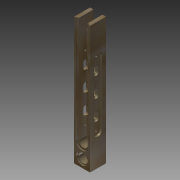
# Autodesk Inventor part: 13_1087_009
Saved by Autodesk Inventor 2014 (Build 180170000, 170)
## iProperties
Created: 2013-08-07
Part Number: 13_1087_009
Material: PVC, hart
Document SubType Name: Modeling
Designer: vogel
Density: 1.4 g/cm^3
Appearance: Sperrholz - verwittert
Author: vogel
Autodesk Inventor part; units mm, degrees
ref_plane "YZ Plane" through (0, 0, 0) normal (1, 0, 0) x (0, 1, 0)
ref_plane "XZ Plane" through (0, 0, 0) normal (0, 1, 0) x (-1, 0, 0)
sketch "Skizze1" plane through (0, 0, 0) normal (0, 0, 1) x (1, 0, 0)
  line L0 (-9.8, 0) -> (9.8, 0) projected
  line L1 (0, -9.8) -> (0, 9.8) projected
  line L2 (-7, 7) -> (7, 7)
  line L3 (7, 7) -> (7, -7)
  line L4 (7, -7) -> (-7, -7)
  line L5 (-7, -7) -> (-7, 7)
  point P0 (0, 0)
  dimension "d0" = 14
  dimension "d1" = 14
  constraints: 8 end point, 2 parallel, 1 horizontal, 1 perpendicular, 2 other
  measures "d0" distance of L2.start L2.end
  measures "d1" distance of L4.end L2.start
extrude "Extrusion1" add sketch "Skizze1" along normal mid plane 82
sketch "Skizze2" plane through (-7, -7, 41) normal (0, -1, 0) x (1, 0, 0)
  line L0 (0, 0) -> (14, 0) projected
  line L1 (0, 0) -> (0, -82) projected
  line L2 (14, -82) -> (0, -82) projected
  line L3 (3, 0) -> (11, 0)
  line L4 (11, 0) -> (11, -12)
  line L5 (11, -12) -> (3, -12)
  line L6 (3, -12) -> (3, 0)
  line L7 (3, -82) -> (11, -82)
  line L8 (11, -82) -> (11, -74)
  line L9 (11, -74) -> (3, -74)
  line L10 (3, -74) -> (3, -82)
  point P0 (7, -41)
  dimension "d6" = 8
  dimension "d7" = 12
  dimension "d8" = 8
  dimension "d9" = 3
  constraints: 16 end point, 4 parallel, 2 collinear, 2 horizontal, 2 perpendicular, 2 point on line
  measures "d6" distance of L4.end L5.end
  measures "d7" distance between parallel lines of L0 L5
  measures "d8" distance between parallel lines of L2 L9
  measures "d9" distance between parallel lines of L1 L6
extrude "Extrusion2" cut sketch "Skizze2" against normal through all
sketch "Skizze3" plane through (-4, -7, 29) normal (0, 0, 1) x (1, 0, 0)
  line L0 (8, 0) -> (8, 14) projected
  line L1 (0, 0) -> (8, 0)
  line L2 (8, 0) -> (8, 8)
  line L3 (8, 8) -> (0, 8)
  line L4 (0, 8) -> (0, 0)
  point P0 (4, 7)
  dimension "d12" = 8
  constraints: 8 end point, 2 parallel, 1 horizontal, 1 perpendicular, 1 point on line
  measures "d12" distance between parallel lines of L3 L1
extrude "Extrusion3" cut sketch "Skizze3" against normal through all
sketch "Skizze4" plane through (-4, 7, 29) normal (0, 0, 1) x (1, 0, 0)
  line L0 (0, 0) -> (8, 0) projected
  line L1 (0, -6) -> (0, 0) projected
  point P0 (4, -7)
  point P1 (4, -4)
  dimension "d15" = 4
  dimension "d16" = 4
  measures "d15" distance from line of L0 point (4, -4)
  measures "d16" distance from line of point (4, -4) L1
hole "Bohrung1" at (0, 3, 29) direction (0, 0, -1) diameter 2.459 depth 7 tip angle 118 thread size "M3x0.5" class "6H" standard "ISO Metric profile"
sketch "Skizze5" plane through (4, 7, -33) normal (0, 0, -1) x (-1, 0, 0)
  line L0 (0, -6) -> (8, -6) projected
  line L1 (8, -6) -> (8, 0) projected
  line L2 (0, 0) -> (8, 0) projected
  line L3 (0, -6) -> (0, 0) projected
  point P0 (4, -7)
extrude "Extrusion4" add sketch "Skizze5" along normal up to surface (8 mm away)
sketch "Skizze6" plane through (0, 0, -41) normal (0, 0, -1) x (-1, 0, 0)
  line L0 (-4, -7) -> (-4, 1) projected
  line L1 (-4, 1) -> (4, 1) projected
  line L2 (4, 1) -> (4, -7) projected
  line L3 (4, -7) -> (7, -7) projected
  line L4 (7, -7) -> (7, 7) projected
  line L5 (7, 7) -> (-7, 7) projected
  line L6 (-7, 7) -> (-7, -7) projected
  line L7 (-7, -7) -> (-4, -7) projected
  point P0 (0, 0)
extrude "Extrusion5" add sketch "Skizze6" along normal blind 30
sketch "Skizze7" plane through (0, 0, -71) normal (0, 0, -1) x (-1, 0, 0)
  line L0 (4, -7) -> (-4, -7)
  line L1 (-4, -7) -> (-4, 1)
  line L2 (-4, 1) -> (4, 1)
  line L3 (4, 1) -> (4, -7)
  point P0 (0, 0)
  constraints: 8 end point, 2 parallel, 1 horizontal, 1 perpendicular
extrude "Extrusion6" add sketch "Skizze7" against normal blind 15
sketch "Skizze8" plane through (-7, -7, -71) normal (0, -1, 0) x (1, 0, 0)
  line L0 (0, 112) -> (0, 0) projected
  line L1 (14, 0) -> (0, 0) projected
  point P0 (7, 71)
  point P1 (7, 7)
  dimension "d30" = 7
  dimension "d31" = 7
  measures "d30" distance from line of point (7, 7) L1
  measures "d31" distance from line of L0 point (7, 7)
hole "Bohrung2" at (0, -7, -64) direction (0, 1, 0) diameter 5 depth 5 tip angle 118
hole "Bohrung3" at (0, -7, -64) direction (0, 1, 0) diameter 8 depth 8 tip angle 118 counterbore diameter 10 counterbore depth 1
fillet "Rundung1" radius 4 2 edges at (4, -3, -56) (-4, -3, -56)
sketch "Skizze9" plane through (7, -7, 41) normal (1, 0, 0) x (0, 0, -1)
  line L0 (0, 14) -> (112, 14) projected
  line L1 (0, 0) -> (0, 14) projected
  line L2 (0, 0) -> (112, 0) projected
  line L3 (27.5, 7) -> (84.5, 7) construction
  line L4 (27.5, 3.5) -> (84.5, 3.5)
  line L5 (84.5, 10.5) -> (27.5, 10.5)
  arc A0 (27.5, 10.5) -> (27.5, 3.5) centre (27.5, 7) ccw
  arc A1 (84.5, 3.5) -> (84.5, 10.5) centre (84.5, 7) ccw
  point P0 (41, 7)
  point P1 (56, 7)
  dimension "d49" = 7
  dimension "d50" = 24
  dimension "d51" = 64
  dimension "d52" = 7
  constraints: 8 end point, 4 point on circle, 4 tangent, 2 centre point, 2 parallel, 1 midpoint
  measures "d49" distance between parallel lines of L5 L4
  measures "d50" distance edge to line of A0 L1
  measures "d52" distance between parallel lines of L3 L2
extrude "Extrusion7" cut sketch "Skizze9" against normal blind 1.5
ref_plane "Arbeitsebene1" through (0, -7, 41) normal (1, 0, 0) x (0, 0, -1)
mirror "Spiegeln1" about plane through (0, -7, 41) normal (1, 0, 0) of "Extrusion7"
sketch "Skizze10" plane through (-4, 7, 29) normal (0, 1, 0) x (1, 0, 0)
  line L0 (8, 0) -> (8, -12) projected
  line L1 (-3, 100) -> (-3, -12) projected
  line L2 (0, -12) -> (-3, -12) projected
  line L3 (4, 55) -> (4, 15.5) construction
  line L4 (0.5, 55) -> (0.5, 15.5)
  line L5 (7.5, 15.5) -> (7.5, 55)
  arc A0 (7.5, 55) -> (0.5, 55) centre (4, 55) ccw
  arc A1 (0.5, 15.5) -> (7.5, 15.5) centre (4, 15.5) ccw
  point P0 (4, 29)
  point P1 (4, 35.25)
  dimension "d55" = 7
  dimension "d57" = 7
  dimension "d58" = 24
  dimension "d59" = 46.5
  constraints: 8 end point, 4 point on circle, 4 tangent, 2 centre point, 2 parallel, 1 midpoint
  measures "d55" distance between parallel lines of L4 L5
  measures "d57" distance between parallel lines of L1 L3
  measures "d58" distance edge to line of A1 L2
extrude "Extrusion8" cut sketch "Skizze10" against normal blind 1.5
sketch "Skizze11" plane through (5.5, -7, 41) normal (1, 0, 0) x (0, 0, -1)
  arc A0 (40.5, 5) -> (40.5, 9) centre (40.5, 7) ccw projected
  line L0 (40.5, 5) -> (36.5, 5) projected
  arc A1 (36.5, 9) -> (36.5, 5) centre (36.5, 7) ccw projected
  line L1 (36.5, 9) -> (40.5, 9) projected
  arc A2 (43.5, 4.5) -> (43.5, 9.5) centre (43.5, 7) ccw projected
  line L2 (43.5, 9.5) -> (33.5, 9.5) projected
  arc A3 (33.5, 9.5) -> (33.5, 4.5) centre (33.5, 7) ccw projected
  line L3 (33.5, 4.5) -> (43.5, 4.5) projected
  line L4 (112, 14) -> (0, 14) projected
  arc A4 (58, 5) -> (58, 9) centre (58, 7) ccw projected
  line L5 (58, 5) -> (54, 5) projected
  arc A5 (54, 9) -> (54, 5) centre (54, 7) ccw projected
  line L6 (54, 9) -> (58, 9) projected
  arc A6 (61, 4.5) -> (61, 9.5) centre (61, 7) ccw projected
  line L7 (61, 9.5) -> (51, 9.5) projected
  arc A7 (51, 9.5) -> (51, 4.5) centre (51, 7) ccw projected
  line L8 (51, 4.5) -> (61, 4.5) projected
  arc A8 (71.5, 9) -> (71.5, 5) centre (71.5, 7) ccw projected
  line L9 (71.5, 9) -> (75.5, 9) projected
  arc A9 (75.5, 5) -> (75.5, 9) centre (75.5, 7) ccw projected
  line L10 (75.5, 5) -> (71.5, 5) projected
  arc A10 (78.5, 4.5) -> (78.5, 9.5) centre (78.5, 7) ccw projected
  line L11 (78.5, 9.5) -> (68.5, 9.5) projected
  arc A11 (68.5, 9.5) -> (68.5, 4.5) centre (68.5, 7) ccw projected
  line L12 (68.5, 4.5) -> (78.5, 4.5) projected
  point P0 (41, 7)
extrude "Extrusion9" cut sketch "Skizze11" against normal through all contours L0 A1 L1 A0 | L5 A5 L6 A4 | L9 A9 L10 A8
sketch "Skizze12" plane through (0, 0, 41) normal (0, 0, 1) x (1, 0, 0)
  line L0 (4, -7) -> (7, -7) projected
  line L1 (5.5, -7) -> (-5.5, -7)
  line L2 (-5.5, -7) -> (-5.5, -6)
  line L3 (-5.5, -6) -> (5.5, -6)
  line L4 (5.5, -6) -> (5.5, -7)
  point P0 (0, 0)
  dimension "d64" = 11
  dimension "d65" = 1
  constraints: 8 end point, 2 parallel, 1 horizontal, 1 midpoint, 1 perpendicular
  measures "d64" distance of L1.start L1.end
  measures "d65" distance between parallel lines of L3 L1
extrude "Extrusion10" cut sketch "Skizze12" against normal blind 98.5
fillet "Rundung2" radius 5 2 edges at (-5.5, -6.5, -57.5) (5.5, -6.5, -57.5)
sketch "Skizze13" plane through (-4, 7, 29) normal (0, 1, 0) x (1, 0, 0)
  arc A0 (2, 42) -> (6, 42) centre (4, 42) ccw projected
  line L0 (2, 42) -> (2, 46) projected
  arc A1 (6, 46) -> (2, 46) centre (4, 46) ccw projected
  line L1 (6, 46) -> (6, 42) projected
  arc A2 (1.5, 39) -> (6.5, 39) centre (4, 39) ccw projected
  line L2 (6.5, 39) -> (6.5, 49) projected
  arc A3 (6.5, 49) -> (1.5, 49) centre (4, 49) ccw projected
  line L3 (1.5, 49) -> (1.5, 39) projected
  arc A4 (6, 28.5) -> (2, 28.5) centre (4, 28.5) ccw projected
  line L4 (6, 28.5) -> (6, 24.5) projected
  arc A5 (2, 24.5) -> (6, 24.5) centre (4, 24.5) ccw projected
  line L5 (2, 24.5) -> (2, 28.5) projected
  arc A6 (1.5, 21.5) -> (6.5, 21.5) centre (4, 21.5) ccw projected
  line L6 (6.5, 21.5) -> (6.5, 31.5) projected
  arc A7 (6.5, 31.5) -> (1.5, 31.5) centre (4, 31.5) ccw projected
  line L7 (1.5, 31.5) -> (1.5, 21.5) projected
  point P0 (4, 29)
extrude "Extrusion11" cut sketch "Skizze13" against normal through all contours L0 A1 L1 A0 | L4 A5 L5 A4
sketch "Skizze14" plane through (7, -7, 41) normal (1, 0, 0) x (0, 0, -1)
  circle A0 centre (27.5, 7) radius 1.2 projected
  circle A1 centre (84.5, 7) radius 1.2 projected
  point P0 (41, 7)
  constraints: 2 coincident
hole "Bohrung4" at (7, 0, 13.5) at (7, 0, -43.5) direction (-1, 0, 0) diameter 1.567 depth 3 tip angle 118 thread size "M2x0.4" class "6H" standard "ISO Metric profile"
sketch "Skizze15" plane through (-4, 7, 29) normal (0, 1, 0) x (1, 0, 0)
  line L0 (0.5, 15.5) -> (0.5, 55) projected
  arc A0 (0.5, 15.5) -> (7.5, 15.5) centre (4, 15.5) ccw projected
  line L1 (7.5, 55) -> (7.5, 15.5) projected
  arc A1 (7.5, 55) -> (0.5, 55) centre (4, 55) ccw projected
  circle A2 centre (4, 15.5) radius 1.2 projected
  circle A3 centre (4, 55) radius 1.2 projected
  point P0 (4, 29)
  constraints: 2 coincident
hole "Bohrung5" at (0, 7, -26) at (0, 7, 13.5) direction (0, -1, 0) diameter 1.567 end through all thread size "M2x0.4" class "6H" standard "ISO Metric profile"
sketch "Skizze16" plane through (-7, -7, 41) normal (-1, 0, 0) x (0, 0, 1)
  arc A0 (-84.5, 10.5) -> (-84.5, 3.5) centre (-84.5, 7) ccw projected
  arc A1 (-27.5, 3.5) -> (-27.5, 10.5) centre (-27.5, 7) ccw projected
  point P0 (-41, 7)
hole "Bohrung6" at (-7, 0, 13.5) at (-7, 0, -43.5) direction (1, 0, 0) diameter 1.567 depth 3 tip angle 118 thread size "M2x0.4" class "6H" standard "ISO Metric profile"
sketch "Skizze17" plane through (0, 1, -52) normal (0, -1, 0) x (1, 0, 0)
  circle A0 centre (0, 11) radius 1.25 projected
  circle A1 centre (0, 71) radius 1.25 projected
  point P0 (0, 52)
hole "Bohrung7" at (0, 1, -41) at (0, 1, 19) direction (0, 1, 0) diameter 1.567 depth 5 tip angle 118 thread size "M2x0.4" class "6H" standard "ISO Metric profile"
hole "Bohrung8" at (0, -7, -64) direction (0, 1, 0) diameter 7.5 end through all
thread "Gewinde1" size "M8x0.5" class "6H" standard "ANSI Metric M Profile" full length
